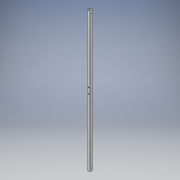
# Autodesk Inventor part: suporte sensores 1m
Saved by Autodesk Inventor 2019.4 (Build 234330000, 330)
## iProperties
Created: 2020-08-25
Part Number: suporte sensores 1m
Material: Alumínio 6061
Document SubType Name: Modeling
Designer: Lattes
Density: 2.7 g/cm^3
Appearance: Alumínio - Polido
Author: Lattes
Autodesk Inventor part; units mm, degrees
ref_plane "YZ Plane" through (0, 0, 0) normal (1, 0, 0) x (0, 1, 0)
ref_plane "XZ Plane" through (0, 0, 0) normal (0, 1, 0) x (-1, 0, 0)
ref_plane "XY Plane" through (0, 0, 0) normal (0, 0, 1) x (1, 0, 0)
sketch "Esboço1" plane through (0, 0, 0) normal (0, 1, 0) x (-1, 0, 0)
  line L0 (0, 0) -> (19.05, 0)
  line L1 (19.05, 0) -> (19.05, -19.05)
  line L2 (19.05, -19.05) -> (0, -19.05)
  line L3 (0, -19.05) -> (0, 0)
  line L4 (17.55, -17.55) -> (17.55, -1.5)
  line L5 (1.5, -1.5) -> (17.55, -1.5)
  line L6 (17.55, -17.55) -> (1.5, -17.55)
  line L7 (1.5, -1.5) -> (1.5, -17.55)
  dimension "d1" = 19.05
  dimension "d2" = 19.05
  dimension "d3" = 19.05
  constraints: 16 end point, 2 perpendicular, 1 horizontal
  measures "d1" distance of L0.start L0.end
  measures "d2" distance of L0.end L1.end
  measures "d3" distance of L1.end L2.end
extrude "Extrusão1" add sketch "Esboço1" along normal blind 1000
sketch "Esboço2" plane through (-19.05, 0, -19.05) normal (0, 0, -1) x (-1, 0, 0)
  point P0 (-19.05, 0)
sketch "Esboço3" plane through (0, 0, 0) normal (0, 0, 1) x (1, 0, 0)
  line L0 (-19.05, 0) -> (0, 0) projected
  line L1 (0, 0) -> (-19.05, 0)
  line L2 (-9.525, 480) -> (-9.525, 520)
  line L3 (-9.525, 500) -> (-9.525, 520.5)
  line L4 (-9.525, 520.5) -> (-9.525, 479.5)
  circle A0 centre (-9.525, 479.5) radius 3.5
  circle A1 centre (-9.525, 520.5) radius 3.5
  dimension "d16" = 40
  dimension "d36" = 20.5
  dimension "d37" = 41
  dimension "d38" = 7
  dimension "d39" = 7
  constraints: 8 end point, 2 centre point, 2 coincident, 2 point on line, 1 collinear, 1 midpoint
  measures "d16" distance of L2.start L2.end
  measures "d36" distance of L3.start L3.end
  measures "d37" distance of L3.end L4.end
  measures "d38" diameter of A0
  measures "d39" diameter of A1
extrude "Extrusão2" cut sketch "Esboço3" against normal blind 20
fillet "Arredondamento1" radius 0.5 4 edges at (0, 500, -19.05) (-19.05, 500, -19.05) (-19.05, 500, 0) (0, 500, 0)
sketch "Esboço5" plane through (0, 0, -0.5) normal (1, 0, 0) x (0, 0, -1)
  line L0 (17.05, 0) -> (1, 0) projected
  circle A0 centre (9.025, 20) radius 2.25
  line L1 (17.05, 1000) -> (1, 1000) projected
  circle A1 centre (9.025, 980) radius 2.25
  point P0 (-0.5, 0)
  dimension "d31" = 4.5
  dimension "d33" = 4.5
  constraints: 2 centre point
  measures "d31" diameter of A0
  measures "d33" diameter of A1
extrude "Extrusão4" cut sketch "Esboço5" against normal blind 20
fillet "Arredondamento2" radius 0.5 4 edges at (-13.025, 479.5, 0) (-13.025, 520.5, 0) (-13.025, 479.5, -19.05) (-13.025, 520.5, -19.05)
